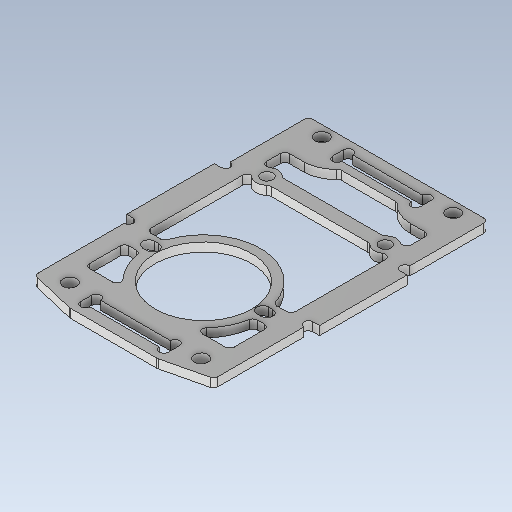
# Autodesk Inventor part: Trunk_horizontal_frame_03
Saved by Autodesk Inventor 2020.4 (Build 244396000, 396)
## iProperties
Created: 2021-09-09
Part Number: Trunk_horizontal_frame_03
Material: アルミニウム 2014-T4
Document SubType Name: Modeling
Designer: Masato Kubotera
Density: 2.8 g/cm^3
Appearance: 滑らか - 淡い灰色
Description: A2017 T2
Author: Masato Kubotera
Autodesk Inventor part; units mm, degrees
ref_plane "YZ Plane" through (0, 0, 0) normal (1, 0, 0) x (0, 1, 0)
ref_plane "XZ Plane" through (0, 0, 0) normal (0, 1, 0) x (-1, 0, 0)
ref_plane "XY Plane" through (0, 0, 0) normal (0, 0, 1) x (1, 0, 0)
sketch "スケッチ1" plane through (0, 0, 0) normal (0, 0, 1) x (1, 0, 0)
  circle A0 centre (0, 0) radius 11
  line L0 (-20.5, -24.5) -> (-22, -24.5)
  line L1 (-22, -24.5) -> (-22, -4.5)
  line L2 (-22, -4.5) -> (-20.5, -4.5)
  circle A1 centre (-13.5, -28) radius 1.35
  arc A2 (-20.5, -26.6) -> (-20.5, -24.5) centre (-20.5, -25.55) ccw
  arc A3 (-20.5, -4.5) -> (-20.5, -2.4) centre (-20.5, -3.45) ccw
  arc A4 (-7.6649, 10.5) -> (-12.9132, 1.5) centre (0, 0) ccw
  arc A5 (-12.52, -3.5) -> (12.52, -3.5) centre (0, 0) ccw
  arc A6 (-11.5, -26.5) -> (-15.5, -26.5) centre (-13.5, -28) ccw
  line L3 (-16.5, 10.5) -> (-7.6649, 10.5)
  line L4 (-16.5, 10.5) -> (-16.5, 1.5)
  line L5 (-16.5, 1.5) -> (-12.9132, 1.5)
  line L6 (-16.5, -3.5) -> (-12.52, -3.5)
  line L7 (-16.5, -3.5) -> (-16.5, -26.5)
  line L8 (-35, -44.5) -> (35, -44.5) construction
  line L9 (35, -44.5) -> (35, -39.5) construction
  line L10 (35, -39.5) -> (-35, -39.5) construction
  line L11 (-35, -39.5) -> (-35, -44.5) construction
  line L12 (-35, -44.5) -> (35, -39.5) construction
  line L13 (35, -44.5) -> (-35, -39.5) construction
  line L14 (-35, -42) -> (35, -42) construction
  line L15 (0, -44.5) -> (0, 20.5) construction
  line L16 (-10, 20.5) -> (10, 20.5)
  line L17 (-20.5, -44.5) -> (20.5, -44.5)
  line L18 (-13.5, -1) -> (0, -1) construction
  line L19 (-13.5, -28) -> (-13.5, -1) construction
  circle A7 centre (-15, -42) radius 1.55
  line L20 (-10, -42) -> (10, -42) construction
  line L21 (10, -42) -> (10, -39.5) construction
  line L22 (-10, -39.5) -> (-10, -42) construction
  line L23 (-10, -42) -> (10, -39.5) construction
  line L24 (10, -42) -> (-10, -39.5) construction
  line L25 (-20.5, -26.6) -> (-20.5, -44.5)
  line L26 (-20.5, -2.4) -> (-20.5, 18)
  line L27 (-20.5, 18) -> (-10, 20.5)
  line L28 (-10.01, -42.01) -> (10.01, -42.01)
  line L29 (10.01, -42.01) -> (10.01, -39.49)
  line L30 (10.01, -39.49) -> (-10.01, -39.49)
  line L31 (-10.01, -39.49) -> (-10.01, -42.01)
  line L32 (-10.01, -42.01) -> (10.01, -39.49) construction
  line L33 (10.01, -42.01) -> (-10.01, -39.49) construction
  line L34 (-10.01, -40.75) -> (10.01, -40.75) construction
  arc A8 (-10.01, -42.01) -> (-7.91, -42.01) centre (-8.96, -42.01) ccw
  arc A9 (-7.91, -39.49) -> (-10.01, -39.49) centre (-8.96, -39.49) ccw
  line L35 (-35, 13) -> (35, 13) construction
  line L36 (35, 13) -> (35, 18) construction
  line L37 (35, 18) -> (-35, 18) construction
  line L38 (-35, 18) -> (-35, 13) construction
  line L39 (-35, 13) -> (35, 18) construction
  line L40 (35, 13) -> (-35, 18) construction
  line L41 (-35, 15.5) -> (35, 15.5) construction
  circle A10 centre (-15, 15.5) radius 1.55
  line L42 (-10, 15.5) -> (10, 15.5) construction
  line L43 (10, 15.5) -> (10, 18) construction
  line L44 (-10, 18) -> (-10, 15.5) construction
  line L45 (-10, 15.5) -> (10, 18) construction
  line L46 (10, 15.5) -> (-10, 18) construction
  line L47 (-10.01, 15.49) -> (10.01, 15.49)
  line L48 (10.01, 15.49) -> (10.01, 18.01)
  line L49 (10.01, 18.01) -> (-10.01, 18.01)
  line L50 (-10.01, 18.01) -> (-10.01, 15.49)
  line L51 (-10.01, 15.49) -> (10.01, 18.01) construction
  line L52 (10.01, 15.49) -> (-10.01, 18.01) construction
  line L53 (-10.01, 16.75) -> (10.01, 16.75) construction
  arc A11 (-10.01, 15.49) -> (-7.91, 15.49) centre (-8.96, 15.49) ccw
  arc A12 (-7.91, 18.01) -> (-10.01, 18.01) centre (-8.96, 18.01) ccw
  line L54 (20.5, -24.5) -> (22, -24.5)
  line L55 (22, -24.5) -> (22, -4.5)
  line L56 (22, -4.5) -> (20.5, -4.5)
  circle A13 centre (13.5, -28) radius 1.35
  arc A14 (20.5, -24.5) -> (20.5, -26.6) centre (20.5, -25.55) ccw
  arc A15 (20.5, -2.4) -> (20.5, -4.5) centre (20.5, -3.45) ccw
  line L57 (16.5, -26.5) -> (15.5, -26.5)
  line L58 (16.5, -3.5) -> (16.5, -26.5)
  arc A16 (15.5, -26.5) -> (11.5, -26.5) centre (13.5, -28) ccw
  arc A17 (12.9132, 1.5) -> (7.6649, 10.5) centre (0, 0) ccw
  line L59 (16.5, 1.5) -> (12.9132, 1.5)
  line L60 (16.5, 10.5) -> (16.5, 1.5)
  line L61 (16.5, 10.5) -> (7.6649, 10.5)
  line L62 (16.5, -3.5) -> (12.52, -3.5)
  circle A18 centre (15, -42) radius 1.55
  line L63 (20.5, -26.6) -> (20.5, -44.5)
  line L64 (20.5, -2.4) -> (20.5, 18)
  line L65 (20.5, 18) -> (10, 20.5)
  arc A19 (7.91, -42.01) -> (10.01, -42.01) centre (8.96, -42.01) ccw
  arc A20 (10.01, -39.49) -> (7.91, -39.49) centre (8.96, -39.49) ccw
  arc A21 (10.01, 18.01) -> (7.91, 18.01) centre (8.96, 18.01) ccw
  arc A22 (7.91, 15.49) -> (10.01, 15.49) centre (8.96, 15.49) ccw
  circle A23 centre (15, 15.5) radius 1.55
  circle A24 centre (-13.5, -1) radius 2.5 construction
  line L66 (-16.5, -26.5) -> (-15.5, -26.5)
  line L67 (-20.5, -28) -> (0, -28) construction
  line L68 (-11.5, -26.5) -> (11.5, -26.5)
  arc A25 (-15.5, -29.5) -> (-11.5, -29.5) centre (-13.5, -28) ccw
  arc A26 (11.5, -29.5) -> (15.5, -29.5) centre (13.5, -28) ccw
  line L69 (16.5, -29.5) -> (15.5, -29.5)
  line L70 (-16.5, -29.5) -> (-15.5, -29.5)
  line L71 (-11.5, -29.5) -> (11.5, -29.5)
  line L72 (-16.5, -29.5) -> (-16.5, -35.0667)
  line L73 (-16.5, -35.0667) -> (-12.0888, -35.0667)
  line L74 (-6.65, -37.7) -> (6.65, -37.7)
  line L75 (-16.5, -31) -> (0, -31) construction
  arc A27 (-6.65, -37.7) -> (-12.0888, -35.0667) centre (-12.0888, -42) ccw
  line L76 (16.5, -35.0667) -> (12.0888, -35.0667)
  arc A28 (12.0888, -35.0667) -> (6.65, -37.7) centre (12.0888, -42) ccw
  line L77 (16.5, -29.5) -> (16.5, -35.0667)
  line L78 (-22, -14.5) -> (-13.5, -14.5) construction
  arc A29 (-12.5, -2.35) -> (-12.5, 0.35) centre (-12.5, -1) ccw
  line L79 (-13.5, -2.35) -> (-12.5, -2.35)
  line L80 (-12.5, 0.35) -> (-13.5, 0.35)
  arc A30 (-13.5, 0.35) -> (-13.5, -2.35) centre (-13.5, -1) ccw
  arc A31 (12.5, 0.35) -> (12.5, -2.35) centre (12.5, -1) ccw
  line L81 (13.5, -2.35) -> (12.5, -2.35)
  line L82 (12.5, 0.35) -> (13.5, 0.35)
  arc A32 (13.5, -2.35) -> (13.5, 0.35) centre (13.5, -1) ccw
  circle A33 centre (-30.4504, -28) radius 2.4 construction
  point P0 (0, -42)
  point P1 (0, -40.75)
  point P2 (0, -42)
  point P3 (0, 15.5)
  point P4 (0, 16.75)
  point P5 (0, 15.5)
  point P6 (0, 15.5)
  point P7 (0, 16.75)
  point P8 (7.91, -42.01)
  point P9 (7.91, 15.49)
  point P10 (7.91, 18.01)
  dimension "d0" = 22
  dimension "d38" = 1.5
  dimension "d39" = 20
  dimension "d151" = 1.05
  dimension "d152" = 1.05
  dimension "d171" = 70
  dimension "d172" = 5
  dimension "d173" = 1
  dimension "d176" = 20
  dimension "d177" = 2.5
  dimension "d178" = 2
  dimension "d179" = 2
  dimension "d180" = 1.05
  dimension "d181" = 0.01
  dimension "d182" = 0.01
  dimension "d183" = 3.1
  dimension "d184" = 70
  dimension "d185" = 5
  dimension "d186" = 20
  dimension "d187" = 2.5
  dimension "d188" = 1.05
  dimension "d189" = 0.01
  dimension "d190" = 0.01
  dimension "d191" = 3.1
  dimension "d192" = 52.5
  dimension "d193" = 2.5
  dimension "d194" = 13
  dimension "d195" = 30
  dimension "d196" = 30
  dimension "d197" = 41
  dimension "d198" = 27
  dimension "d199" = 2.7
  dimension "d200" = 2.5
  dimension "d201" = 2.5
  dimension "d202" = 4
  dimension "d204" = 5
  dimension "d205" = 3
  dimension "d206" = 3
  dimension "d207" = 4.0667
  dimension "d208" = 6.7
  dimension "d211" = 13.3
  dimension "d213" = 2.7
  dimension "d214" = 27
  dimension "d215" = 1
  dimension "d216" = 4.8
  dimension "d217" = 13.5
  constraints: 166 end point, 50 point on circle, 39 horizontal alignment, 34 centre point, 28 midpoint, 24 point on line, 16 horizontal, 13 equal radius, 11 parallel, 11 perpendicular, 10 symmetric about line, 9 tangent, 6 vertical, 4 coincident, 4 collinear, 3 concentric, 15 other
  measures "d0" diameter of A0
  measures "d38" distance of L0.start L0.end
  measures "d39" distance of L0.end L1.end
  measures "d151" radius of A2
  measures "d152" radius of A3
  measures "d171" distance of L10.end L9.end
  measures "d172" distance of L9.end L8.end
  measures "d173" distance of A4.centre L18.end
  measures "d176" distance of L22.start L21.end
  measures "d177" distance of L21.end L20.end
  measures "d178" radial gap between concentric circles of A0 A5
  measures "d179" radial gap between concentric circles of A0 A4
  measures "d180" radius of A8
  measures "d181" horizontal distance of L22.start L30.end
  measures "d182" horizontal distance of L22.start L30.end
  measures "d183" diameter of A7
  measures "d184" distance of L37.end L36.end
  measures "d185" distance of L36.end L35.end
  measures "d186" distance of L46.end L43.end
  measures "d187" distance of L43.end L42.end
  measures "d188" radius of A11
  measures "d189" horizontal distance of L46.end L49.end
  measures "d190" horizontal distance of L46.end L49.end
  measures "d191" diameter of A10
  measures "d192" distance of L35.start L10.end
  measures "d193" distance from line of point (0, 20.5) L37
  measures "d194" distance from line of L35 point (0, 0)
  measures "d195" distance of A18.centre A7.centre
  measures "d196" distance of A23.centre A10.centre
  measures "d197" distance of L17.end L17.start
  measures "d198" distance of A16.centre A1.centre
  measures "d199" diameter of A1
  measures "d200" radius of A6
  measures "d201" distance between parallel lines of L35 L3
  measures "d202" horizontal distance of L4.start L26.end
  measures "d204" diameter of A24
  measures "d205" distance of L7.end L70.start
  measures "d206" distance from line of A1.centre L75
  measures "d207" distance of L72.end L75.start
  measures "d208" distance between parallel lines of L75 L74
  measures "d211" distance of L74.start L74.end
  measures "d213" diameter of A29
  measures "d214" distance of L19.start L18.start
  measures "d215" distance of A24.centre A29.centre
  measures "d216" diameter of A33
  measures "d217" vertical distance of A33.centre L78.start
extrude "押し出し1" add sketch "スケッチ1" along normal blind 2
fillet "フィレット1" radius 1 6 edges at (-20.5, -44.5, 1) (20.5, -44.5, 1) (20.5, 18, 1) (-20.5, 18, 1) (-10, 20.5, 1) (10, 20.5, 1)
fillet "フィレット2" radius 1 27 edges at (-16.5, -35.0667, 1) (-6.65, -37.7, 1) (6.65, -37.7, 1) (16.5, -35.0667, 1) (16.5, -29.5, 1) (16.5, -26.5, 1) (11.5, -26.5, 1) (11.5, -29.5, 1) (-11.5, -26.5, 1) (-11.5, -29.5, 1) (-15.5, -26.5, 1) (-15.5, -29.5, 1) (-16.5, -29.5, 1) (-16.5, -26.5, 1) (-16.5, -3.5, 1) (-12.52, -3.5, 1) (-12.9132, 1.5, 1) (-16.5, 1.5, 1) (12.52, -3.5, 1) (16.5, -3.5, 1) (16.5, 1.5, 1) (12.9132, 1.5, 1) (-7.6649, 10.5, 1) (-16.5, 10.5, 1) (7.6649, 10.5, 1) (16.5, 10.5, 1) (15.5, -29.5, 1)
